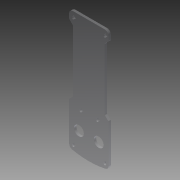
# Autodesk Inventor part: Top Plate
Saved by Autodesk Inventor 2015 (Build 190159000, 159)
## iProperties
Created: 2016-02-20
Part Number: Top Plate
Material: Polycarbonate, Clear
Document SubType Name: Modeling
Designer: 23902
Density: 1.2 g/cm^3
Appearance: Polycarbonate - Clear
Mass: 23.5455 g
Surface Area: 147.116 cm^2
Volume: 19.6213 cm^3
Author: 23902
Autodesk Inventor part; units mm, degrees
ref_plane "YZ Plane" through (0, 0, 0) normal (1, 0, 0) x (0, 1, 0)
ref_plane "XZ Plane" through (0, 0, 0) normal (0, 1, 0) x (-1, 0, 0)
ref_plane "XY Plane" through (0, 0, 0) normal (0, 0, 1) x (1, 0, 0)
sketch "Sketch1" plane through (0, 0, 0) normal (0, 1, 0) x (-1, 0, 0)
  circle A0 centre (-20, 47.5) radius 1.6
  circle A1 centre (20, 47.5) radius 1.6
  circle A2 centre (-20, -92.5) radius 1.6
  circle A3 centre (20, -92.5) radius 1.6
  line L0 (20, 55) -> (-20, 55)
  line L1 (-25, -92.5) -> (-25, -92.5494)
  line L2 (25, -92.5) -> (25, -92.5494)
  arc A4 (-21.0561, -97.4366) -> (21.0561, -97.4366) centre (0, 0) ccw
  arc A5 (21.0561, -97.4366) -> (25, -92.5494) centre (20, -92.5494) ccw
  arc A6 (-25, -92.5494) -> (-21.0561, -97.4366) centre (-20, -92.5494) ccw
  arc A7 (-20, 55) -> (-25, 50) centre (-20, 50) ccw
  arc A8 (25, 50) -> (20, 55) centre (20, 50) ccw
  circle A9 centre (-10.5, -49.6569) radius 1.65
  circle A10 centre (10.5, -49.6569) radius 1.6
  circle A11 centre (-12.5, -72.5) radius 6.25
  circle A12 centre (12.5, -72.5) radius 6.25
  line L3 (-20, 38.3431) -> (-20, -38)
  line L4 (-24.4142, 43.5858) -> (-20.5858, 39.7574)
  line L5 (-24.4142, -43.2426) -> (-20.5858, -39.4142)
  line L6 (-25, -92.5494) -> (-25, -44.6569)
  line L7 (-25, 45) -> (-25, 50)
  line L8 (20, 38.3431) -> (20, -38)
  line L9 (24.4142, 43.5858) -> (20.5858, 39.7574)
  line L10 (24.4142, -43.2426) -> (20.5858, -39.4142)
  line L11 (25, -92.5494) -> (25, -44.6569)
  line L12 (25, 45) -> (25, 50)
  arc A13 (-25, 45) -> (-24.4142, 43.5858) centre (-23, 45) ccw
  arc A14 (-20, 38.3431) -> (-20.5858, 39.7574) centre (-22, 38.3431) ccw
  arc A15 (-20.5858, -39.4142) -> (-20, -38) centre (-22, -38) ccw
  arc A16 (-24.4142, -43.2426) -> (-25, -44.6569) centre (-23, -44.6569) ccw
  arc A17 (25, -44.6569) -> (24.4142, -43.2426) centre (23, -44.6569) ccw
  arc A18 (20, -38) -> (20.5858, -39.4142) centre (22, -38) ccw
  arc A19 (20.5858, 39.7574) -> (20, 38.3431) centre (22, 38.3431) ccw
  arc A20 (24.4142, 43.5858) -> (25, 45) centre (23, 45) ccw
  constraints: 26 end point, 26 point on circle, 21 centre point, 2 point on line
extrude "Extrusion1" add sketch "Sketch1" along normal blind 3
body "Solid1"
